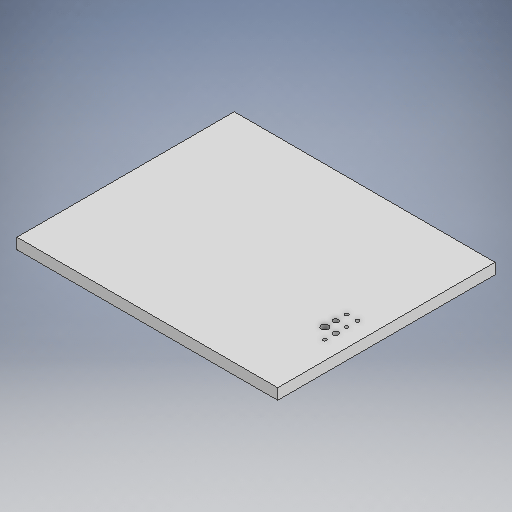
# Autodesk Inventor part: Concrete Pad
Saved by Autodesk Inventor 2025.3 (Build 293356000, 356)
## iProperties
Created: 2025-11-10
Part Number: Concrete Pad
Material: Generic
Document SubType Name: Modeling
Designer: sonata
Density: 1 g/cm^3
Appearance: Default
Author: sonata
Autodesk Inventor part; units mm, degrees
ref_plane "YZ Plane" through (0, 0, 0) normal (1, 0, 0) x (0, 1, 0)
ref_plane "XZ Plane" through (0, 0, 0) normal (0, 1, 0) x (-1, 0, 0)
ref_plane "XY Plane" through (0, 0, 0) normal (0, 0, 1) x (1, 0, 0)
sketch "Sketch1" plane through (0, 0, 0) normal (0, 1, 0) x (-1, 0, 0)
  line L0 (0, 0) -> (3657.6, 0)
  line L1 (3657.6, 0) -> (3657.6, -3048)
  line L2 (3657.6, -3048) -> (0, -3048)
  line L3 (0, -3048) -> (0, 0)
  dimension "d0" = 3657.6
  dimension "d1" = 3048
  constraints: 8 end point, 2 parallel, 1 horizontal, 1 perpendicular
  measures "d0" distance of L1.end L2.end
  measures "d1" distance of L0.end L1.end
extrude "Extrusion1" add sketch "Sketch1" along normal blind 152.4
sketch "Sketch2" plane through (0, 152.4, 0) normal (0, 1, 0) x (1, 0, 0)
  circle A0 centre (-254, 1371.6) radius 25.4
  circle A1 centre (-254, 1219.2) radius 25.4
  circle A2 centre (-254, 1066.8) radius 38.1
  circle A3 centre (-406.4, 1066.8) radius 50.8
  circle A4 centre (-406.4, 1219.2) radius 38.1
  circle A5 centre (-406.4, 1371.6) radius 25.4
  line L0 (0, 0) -> (0, 3048) projected
  line L1 (0, 3048) -> (-3657.6, 3048) projected
  circle A6 centre (-254, 914.4) radius 25.4
  dimension "d5" = 76.2
  dimension "d6" = 50.8
  dimension "d7" = 50.8
  dimension "d8" = 101.6
  dimension "d9" = 76.2
  dimension "d10" = 50.8
  dimension "d11" = 152.4
  dimension "d12" = 152.4
  dimension "d13" = 254
  dimension "d14" = 152.4
  dimension "d15" = 1676.4
  dimension "d20" = 50.8
  dimension "d21" = 152.4
  constraints: 7 centre point, 5 vertical alignment, 3 horizontal alignment
  measures "d5" diameter of A2
  measures "d6" diameter of A1
  measures "d7" diameter of A0
  measures "d8" diameter of A3
  measures "d9" diameter of A4
  measures "d10" diameter of A5
  measures "d11" distance of A4.centre A3.centre
  measures "d12" distance of A5.centre A4.centre
  measures "d13" distance from line of L0 A2.centre
  measures "d14" distance of A2.centre A3.centre
  measures "d15" distance from line of L1 A0.centre
  measures "d20" diameter of A6
  measures "d21" distance of A2.centre A6.centre
extrude "Extrusion2" cut sketch "Sketch2" against normal through all
body "Solid1"
